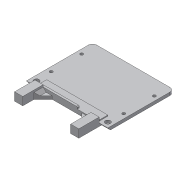
# Autodesk Inventor part: Grundplatte_zerlegt
Saved by Autodesk Inventor 2013 (Build 170138000, 138)
## iProperties
Created: 2013-06-29
Part Number: Grundplatte_zerlegt
Material: Allgemein
Document SubType Name: Modeling
Designer: Harald
Density: 1 g/cm^3
Author: Harald
Autodesk Inventor part; units mm, degrees
ref_plane "YZ Plane" through (0, 0, 0) normal (1, 0, 0) x (0, 1, 0)
ref_plane "XZ Plane" through (0, 0, 0) normal (0, 1, 0) x (-1, 0, 0)
ref_plane "XY Plane" through (0, 0, 0) normal (0, 0, 1) x (1, 0, 0)
sketch "Skizze1" plane through (0, 0, 0) normal (0, 0, 1) x (1, 0, 0)
  line L0 (0, 0) -> (80, 0)
  line L1 (80, 0) -> (80, 65)
  line L2 (80, 65) -> (0, 65)
  line L3 (0, 65) -> (0, 0)
  dimension "d0" = 80
  dimension "d1" = 65
  constraints: 8 end point, 1 horizontal, 1 parallel, 1 perpendicular, 1 vertical
  measures "d0" distance of L2.end L1.end
  measures "d1" distance of L0.end L1.end
extrude "Extrusion2" add sketch "Skizze1" along normal blind 3
sketch "Skizze5" plane through (0, 0, 0) normal (0, -1, 0) x (1, 0, 0)
  line L0 (0, 0) -> (0, 3) projected
  line L1 (8.5, 8) -> (16.5, 8)
  line L2 (16.5, 8) -> (16.5, 0)
  line L3 (16.5, 0) -> (8.5, 0)
  line L4 (8.5, 0) -> (8.5, 8)
  line L5 (63.5, 8) -> (71.5, 8)
  line L6 (71.5, 8) -> (71.5, 0)
  line L7 (71.5, 0) -> (63.5, 0)
  line L8 (63.5, 0) -> (63.5, 8)
  line L9 (0, 0) -> (80, 0) projected
  dimension "d105" = 8
  dimension "d108" = 63
  dimension "d109" = 8.5
  dimension "d112" = 8
  constraints: 16 end point, 4 parallel, 2 collinear, 2 equal length, 2 horizontal, 2 perpendicular
  measures "d105" distance between parallel lines of L2 L4
  measures "d108" distance between parallel lines of L6 L4
  measures "d109" distance between parallel lines of L4 L0
  measures "d112" distance between parallel lines of L3 L1
extrude "Extrusion5" add sketch "Skizze5" along normal blind 20
chamfer "Fase3" distance 9 angle 45 1 edges at (16.5, 0, 1.5)
chamfer "Fase4" distance 9 angle 45 1 edges at (63.5, 0, 1.5)
chamfer "Fase5" distance 3 angle 45 1 edges at (63.5, -4.5, 3)
chamfer "Fase6" distance 3 angle 45 1 edges at (16.5, -4.5, 3)
fillet "Rundung17" radius 4 2 edges at (0, 65, 1.5) (80, 65, 1.5)
sketch "Skizze13" plane through (0, 0, 3) normal (0, 0, 1) x (1, 0, 0)
  line L0 (10, 10) -> (70, 10)
  line L1 (70, 10) -> (70, 0)
  line L2 (70, 0) -> (10, 0)
  line L3 (10, 0) -> (10, 10)
  line L4 (0, 0) -> (8.5, 0) projected
  line L5 (80, 0) -> (80, 61) projected
  dimension "d0" = 80
  dimension "d257" = 60
  dimension "d258" = 10
  dimension "d259" = 10
  constraints: 8 end point, 2 parallel, 1 collinear, 1 horizontal, 1 perpendicular
  measures "d257" distance between parallel lines of L1 L3
  measures "d258" distance between parallel lines of L5 L1
  measures "d259" distance between parallel lines of L2 L0
extrude "Extrusion13" add sketch "Skizze13" along normal blind 1
sketch "Skizze15" plane through (0, 0, 4) normal (0, 0, 1) x (1, 0, 0)
  line L0 (10, 2) -> (50, 2)
  line L1 (50, 2) -> (50, 0)
  line L2 (50, 0) -> (10, 0)
  line L3 (10, 0) -> (10, 2)
  line L4 (0, 61) -> (0, 0) projected
  line L5 (0, 0) -> (8.5, 0) projected
  dimension "d189" = 40
  dimension "d190" = 2
  dimension "d191" = 10
  constraints: 8 end point, 2 parallel, 1 collinear, 1 horizontal, 1 perpendicular
  measures "d189" distance of L1.end L2.end
  measures "d190" distance of L0.end L1.end
  measures "d191" distance between parallel lines of L4 L3
extrude "Extrusion15" add sketch "Skizze15" along normal blind 2
fillet "Rundung19" radius 1 1 edges at (50, 1, 6)
chamfer "Fase13" distance 2.9999 angle 40 1 edges at (75.75, 0, 0) measured on face at (77.1667, 0, 2)
chamfer "Fase14" distance 2.9999 angle 40 1 edges at (4.25, 0, 0) measured on face at (2.8333, 0, 1)
hole "Bohrung5" at (5, 5, 3) direction (0, 0, -1) diameter 5 end through all
hole "Bohrung6" at (75, 5, 3) direction (0, 0, -1) diameter 5 end through all
hole "Bohrung7" at (4.35, 20, 3) direction (0, 0, -1) diameter 3 end through all
hole "Bohrung8" at (4.35, 50, 3) direction (0, 0, -1) diameter 3 end through all
hole "Bohrung9" at (75.65, 20, 3) direction (0, 0, -1) diameter 3 end through all
hole "Bohrung10" at (75.65, 50, 3) direction (0, 0, -1) diameter 3 end through all
chamfer "Fase16" distance 2 angle 45 1 edges at (65.75, 0, 4)
